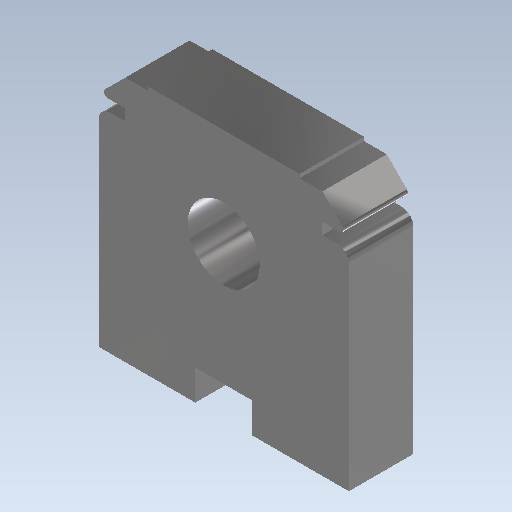
# Autodesk Inventor part: Holder
Saved by Autodesk Inventor 2021.3 (Build 253353000, 353)
## iProperties
Created: 2021-06-01
Part Number: Holder
Material: Steel, Carbon
Document SubType Name: Modeling
Designer: vivek
Density: 7.87 g/cm^3
Appearance: Semi-Polished
Author: vivek
Autodesk Inventor part; units mm, degrees
note: some values were not read from the file. Chosen so that the rebuilt part matches the saved one: sketch regions of "Extrusion2".
ref_plane "YZ Plane" through (0, 0, 0) normal (1, 0, 0) x (0, 1, 0)
ref_plane "XZ Plane" through (0, 0, 0) normal (0, 1, 0) x (-1, 0, 0)
ref_plane "XY Plane" through (0, 0, 0) normal (0, 0, 1) x (1, 0, 0)
sketch "Sketch2" plane through (0, 0, 0) normal (0, 0, 1) x (1, 0, 0)
  line L0 (33, -33) -> (-33, -33)
  line L1 (-33, -33) -> (-33, 33)
  line L2 (-33, 33) -> (33, 33)
  line L3 (33, 33) -> (33, -33)
  line L4 (0, 0) -> (0, 20.7499)
  line L5 (0, 0) -> (18.2964, 0)
  point P0 (0, 33)
  point P1 (33, 0)
  dimension "d17" = 66
  dimension "d18" = 66
  constraints: 12 end point, 3 parallel, 2 midpoint, 2 perpendicular, 2 point on line, 1 horizontal
  measures "d17" distance of L1.end L2.end
  measures "d18" distance of L0.end L1.end
extrude "Extrusion1" add sketch "Sketch2" along normal blind 17
sketch "Sketch3" plane through (0, 0, 0) normal (0, 0, -1) x (-1, 0, 0)
  line L0 (33, -33) -> (33, 33) projected
  line L1 (33, 33) -> (-33, 33) projected
  line L2 (-33, 33) -> (-33, -33) projected
  line L3 (20, 32) -> (-20, 32)
  line L4 (-20, 32) -> (-20, 33)
  line L5 (-20, 33) -> (20, 33)
  line L6 (20, 33) -> (20, 32)
  line L7 (-20, 32) -> (-33, 32)
  line L8 (20, 32) -> (33, 32)
  point P0 (0, 0)
  point P1 (0, 33)
  dimension "d21" = 40
  dimension "d22" = 1
  constraints: 12 end point, 3 perpendicular, 2 midpoint, 2 parallel, 2 point on line, 1 horizontal
  measures "d21" distance of L4.end L5.end
  measures "d22" distance of L3.end L4.end
extrude "Extrusion2" cut sketch "Sketch3" against normal through all contours L8 L6 L1 L0 | L7 L2 L1 L4
chamfer "Chamfer1" distance 7 angle 45 2 edges at (33, 32, 8.5) (-33, 32, 8.5)
sketch "Sketch4" plane through (0, 0, 0) normal (0, 0, -1) x (-1, 0, 0)
  line L0 (-33, 25) -> (-33, -33) projected
  line L1 (33, -33) -> (33, 25) projected
  line L2 (33, 25) -> (26, 25)
  line L3 (26, 25) -> (26, 22)
  line L4 (26, 22) -> (33, 22)
  line L5 (-33, 25) -> (-26, 25)
  line L6 (-26, 25) -> (-26, 22)
  line L7 (-26, 22) -> (-33, 22)
  point P0 (0, 0)
  dimension "d28" = 7
  dimension "d29" = 3
  dimension "d30" = 7
  dimension "d31" = 3
  constraints: 12 end point, 5 perpendicular, 2 point on line, 1 parallel
  measures "d28" distance of L1.end L2.end
  measures "d29" distance of L2.end L3.end
  measures "d30" distance of L0.start L5.end
  measures "d31" distance of L5.end L6.end
extrude "Extrusion3" cut sketch "Sketch4" against normal through all
fillet "Fillet1" radius 1 2 edges at (-33, 25, 8.5) (33, 25, 8.5)
fillet "Fillet2" radius 3 2 edges at (33, 22, 8.5) (-33, 22, 8.5)
sketch "Sketch5" plane through (0, 0, 0) normal (0, 0, -1) x (-1, 0, 0)
  line L0 (-33, -33) -> (33, -33) projected
  line L1 (7.5, -33) -> (-7.5, -33)
  line L2 (-7.5, -33) -> (-7.5, -25)
  line L3 (-7.5, -25) -> (7.5, -25)
  line L4 (7.5, -25) -> (7.5, -33)
  point P0 (0, 0)
  point P1 (0, -33)
  dimension "d36" = 15
  dimension "d37" = 8
  constraints: 8 end point, 2 midpoint, 2 parallel, 1 horizontal, 1 perpendicular
  measures "d36" distance of L2.end L3.end
  measures "d37" distance of L1.end L2.end
extrude "Extrusion4" cut sketch "Sketch5" against normal through all
sketch "Sketch6" plane through (0, 0, 0) normal (0, 0, -1) x (-1, 0, 0)
  line L0 (33, -33) -> (33, 19) projected
  line L1 (20, 33) -> (-20, 33) projected
  circle A0 centre (0, 7) radius 9.5
  point P0 (0, 0)
  dimension "d40" = 19
  dimension "d41" = 26
  dimension "d42" = 33
  constraints: 1 centre point
  measures "d40" diameter of A0
  measures "d41" distance from line of L1 A0.centre
  measures "d42" distance from line of L0 A0.centre
extrude "Extrusion5" cut sketch "Sketch6" against normal through all
body "Solid1"
